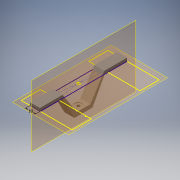
# Autodesk Inventor part: servo_bracket_holder
Saved by Autodesk Inventor 2018 (Build 220112000, 112)
## iProperties
Created: 2018-03-19
Part Number: servo_bracket_holder
Material: Generic
Document SubType Name: Modeling
Designer: erwin
Density: 1 g/cm^3
Appearance: Default
Author: erwin
Autodesk Inventor part; units mm, degrees
ref_plane "YZ Plane" through (0, 0, 0) normal (1, 0, 0) x (0, 1, 0)
ref_plane "XZ Plane" through (0, 0, 0) normal (0, 1, 0) x (-1, 0, 0)
ref_plane "XY Plane" through (0, 0, 0) normal (0, 0, 1) x (1, 0, 0)
ref_plane "Work Plane1" through (0, 0, 0) normal (0, 0, 1) x (1, 0, 0)
sketch "Sketch1" plane through (0, 0, 0) normal (0, 0, 1) x (1, 0, 0)
  circle A0 centre (-32.16, 25) radius 1.5 projected
  line L0 (-46.16, -18.25) -> (4.84, -18.25) projected
  line L1 (4.84, -18.25) -> (4.84, 0.75) projected
  line L2 (4.84, 0.75) -> (-46.16, 0.75) projected
  line L3 (-46.16, -18.25) -> (-46.16, 0.75) projected
  line L4 (4.84, 68.25) -> (-46.16, 68.25) projected
  line L5 (-46.16, 68.25) -> (-46.16, 49.25) projected
  line L6 (-46.16, 49.25) -> (4.84, 49.25) projected
  line L7 (4.84, 68.25) -> (4.84, 49.25) projected
  line L8 (-37.16, 68.25) -> (-27.16, 68.25)
  line L9 (-27.16, 68.25) -> (-27.16, -18.25)
  line L10 (-27.16, -18.25) -> (-37.16, -18.25)
  line L11 (-37.16, -18.25) -> (-37.16, 68.25)
  line L12 (-37.16, 68.25) -> (-27.16, -18.25) construction
  line L13 (-27.16, 68.25) -> (-37.16, -18.25) construction
  point P0 (0, 0)
  dimension "d0" = 10
  constraints: 12 end point, 2 midpoint, 2 parallel, 1 horizontal, 1 perpendicular, 1 point on line
  measures "d0" distance of L9.end L10.end
ref_plane "Work Plane3" through (-27.16, 68.25, 0) normal (1, 0, 0) x (0, -1, 0)
ref_plane "Work Plane2" through (4.84, 54, -29.8) normal (1, 0, 0) x (0, -1, 0)
sketch "Sketch2" plane through (-27.16, 68.25, 0) normal (1, 0, 0) x (0, -1, 0)
  line L0 (58.4964, 22.9) -> (28.0036, 22.9) projected
  line L1 (65, 22.8) -> (65, 15.8) projected
  line L2 (86.7048, 0.0852) -> (64.4463, 0.0852)
  line L3 (64.4463, 0.0852) -> (64.4463, -2.9148)
  line L4 (64.4463, -2.9148) -> (86.7048, -2.9148)
  line L5 (86.7048, -2.9148) -> (86.7048, 0.0852)
  line L6 (43.25, 22.9) -> (52.25, 22.9)
  line L7 (52.25, 22.9) -> (52.25, 18.9)
  line L8 (52.25, 18.9) -> (43.25, 18.9)
  line L9 (43.25, 18.9) -> (43.25, 22.9)
  line L10 (64.4463, 0.0852) -> (52.25, 22.9)
  line L11 (50.14, 18.9) -> (64.0461, -2.9148)
  line L12 (64.0461, -2.9148) -> (64.4463, -2.9148)
  point P0 (68.25, 0)
  dimension "d1" = 3
  dimension "d2" = 9
  dimension "d3" = 4
  constraints: 22 end point, 4 parallel, 3 horizontal, 2 perpendicular, 1 equal length, 1 midpoint, 1 point on line
  measures "d1" distance of L3.end L2.end
  measures "d2" distance of L7.end L8.end
  measures "d3" distance of L6.end L7.end
extrude "Extrusion1" add sketch "Sketch2" against normal blind 10
mirror "Mirror1" about plane through (-27.16, 25, -18.9) normal (0, 1, 0) of "Extrusion1"
sketch "Sketch3" plane through (-37.16, 18.11, -18.9) normal (0, 0, 1) x (1, 0, 0)
  circle A0 centre (5, 6.89) radius 1.5 projected
  point P0 (37.16, -18.11)
  constraints: 1 coincident
hole "Hole1" at (-32.16, 25, -18.9) direction (0, 0, -1) diameter 3 end through all counterbore diameter 7 counterbore depth 0.5
body "Solid1"
